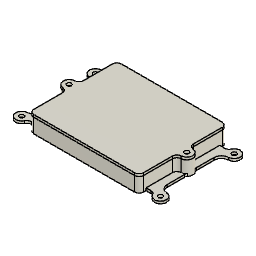
bat case v4 (Autodesk Fusion 360 design; units mm, degrees)
Autodesk Fusion 360 part; units mm, degrees
sketch "Sketch1" plane through (0, 0, 0) normal (0, 0, 1) x (1, 0, 0)
  line L0 (35.1, 27.7) -> (-35.1, 27.7)
  line L1 (-35.1, 27.7) -> (-35.1, -27.7)
  line L2 (-35.1, -27.7) -> (35.1, -27.7)
  line L3 (35.1, -27.7) -> (35.1, 27.7)
  line L4 (35.1, 27.7) -> (-35.1, -27.7) construction
  line L5 (-35.1, 27.7) -> (35.1, -27.7) construction
  circle A0 centre (-46.4, 24.65) radius 1.5
  circle A1 centre (-46.4, -24.65) radius 1.5
  line L6 (-40.0754, -24.65) -> (-36.7, -24.65)
  line L7 (-40.0754, 24.65) -> (-36.7, 24.65)
  arc A2 (-46.6015, -20.6551) -> (-42.786, -26.3643) centre (-46.4, -24.65) ccw
  arc A3 (-42.786, 26.3643) -> (-46.6015, 20.6551) centre (-46.4, 24.65) ccw
  arc A4 (-42.786, 26.3643) -> (-40.0754, 24.65) centre (-40.0754, 27.65) ccw
  arc A5 (-41.8533, 15.6614) -> (-46.6015, 20.6551) centre (-46.8533, 15.6614) ccw
  arc A6 (-46.6015, -20.6551) -> (-41.8533, -15.6614) centre (-46.8533, -15.6614) ccw
  arc A7 (-40.0754, -24.65) -> (-42.786, -26.3643) centre (-40.0754, -27.65) ccw
  line L8 (36.7, -29.3) -> (36.7, 29.3)
  line L9 (36.7, 29.3) -> (-36.7, 29.3)
  line L10 (-36.7, 29.3) -> (-36.7, -29.3)
  line L11 (-36.7, -29.3) -> (36.7, -29.3)
  line L12 (-36.7, 0) -> (-41.8533, 0) construction
  circle A8 centre (-39.2766, 0) radius 1.5
  line L13 (-41.8533, -15.6614) -> (-41.8533, -3.88)
  line L14 (-41.8533, 3.88) -> (-41.8533, 15.6614)
  arc A9 (-42.3277, 2.5867) -> (-42.3277, -2.5867) centre (-39.2766, 0) ccw
  arc A10 (-41.8533, -3.88) -> (-42.3277, -2.5867) centre (-43.8533, -3.88) ccw
  arc A11 (-42.3277, 2.5867) -> (-41.8533, 3.88) centre (-43.8533, 3.88) ccw
  dimension "d1" = 70.2
  dimension "d2" = 55.4
  dimension "d3" = 3
  dimension "d7" = 3
  dimension "d8" = 49.3
  dimension "d9" = 8
  dimension "d10" = 8
  dimension "d11" = 3
  dimension "d12" = 5
  dimension "d13" = 5
  dimension "d14" = 3
  dimension "d15" = 1.6
  dimension "d16" = 3
  dimension "d17" = 8
  dimension "d18" = 2
  dimension "d19" = 2
  constraint horizontal L0
  constraint perpendicular L0 L1
  constraint parallel L0 L2
  constraint parallel L1 L3
  constraint coincident L4 origin
  constraint coincident L5 origin
  constraint concentric A0 A3
  constraint concentric A1 A2
  constraint vertical L13
  constraint perpendicular L1 L6
  constraint perpendicular L1 L7
  constraint tangent L7 A4
  constraint tangent A3 A4
  constraint tangent A5 L13
  constraint tangent A3 A5
  constraint tangent A6 L13
  constraint tangent A2 A6
  constraint tangent L6 A7
  constraint tangent A2 A7
  constraint coincident L10 L7.end
  constraint coincident L10 L6.end
  constraint midpoint L10 L12.start
  constraint perpendicular L12 L13
  constraint midpoint L12 A8.centre
  constraint concentric A8 A9
  constraint collinear L13 L14
  constraint tangent L13 A10
  constraint tangent A9 A10
  constraint tangent L14 A11
  constraint tangent A9 A11
  measures "d1" distance of L1.end L2.end
  measures "d2" distance of L0.end L1.end
  measures "d3" diameter of A0
  measures "d7" diameter of A1
  measures "d8" distance of A0.centre A1.centre
  measures "d9" diameter of A3
  measures "d10" diameter of A2
  measures "d11" radius of A4
  measures "d12" radius of A5
  measures "d13" radius of A6
  measures "d14" radius of A7
  measures "d16" diameter of A8
  measures "d17" diameter of A9
  measures "d18" radius of A10
  measures "d19" radius of A11
extrude "Extrude1" add sketch "Sketch1" along normal blind 1.6 contours L0 L1 L2 L3 | A0 | A1 | L6 L7 A2 A3 A4 A5 A6 A7 L10 L13 L14 A9 A10 A11 | L8 L9 L10 L11 | A8 makes body 1
sketch "Sketch2" plane through (0, 0, 1.6) normal (0, 0, 1) x (-1, 0, 0)
  arc A0 (46.6015, 20.6551) -> (42.786, 26.3643) centre (46.4, 24.65) ccw
  arc A1 (40.0754, 24.65) -> (42.786, 26.3643) centre (40.0754, 27.65) ccw
  line L0 (40.0754, 24.65) -> (36.7, 24.65)
  line L1 (36.7, 24.65) -> (36.7, 29.3)
  line L2 (36.7, 29.3) -> (-36.7, 29.3)
  line L3 (-36.7, 29.3) -> (-36.7, -29.3)
  line L4 (-36.7, -29.3) -> (36.7, -29.3)
  line L5 (36.7, -29.3) -> (36.7, -24.65)
  line L6 (36.7, -24.65) -> (40.0754, -24.65)
  arc A2 (42.786, -26.3643) -> (40.0754, -24.65) centre (40.0754, -27.65) ccw
  arc A3 (42.786, -26.3643) -> (46.6015, -20.6551) centre (46.4, -24.65) ccw
  arc A4 (41.8533, -15.6614) -> (46.6015, -20.6551) centre (46.8533, -15.6614) ccw
  line L7 (41.8533, -15.6614) -> (41.8533, -3.88)
  arc A5 (42.3277, -2.5867) -> (41.8533, -3.88) centre (43.8533, -3.88) ccw
  arc A6 (42.3277, -2.5867) -> (42.3277, 2.5867) centre (39.2766, 0) ccw
  arc A7 (41.8533, 3.88) -> (42.3277, 2.5867) centre (43.8533, 3.88) ccw
  line L8 (41.8533, 3.88) -> (41.8533, 15.6614)
  arc A8 (46.6015, 20.6551) -> (41.8533, 15.6614) centre (46.8533, 15.6614) ccw
  line L9 (35.1, 27.7) -> (-35.1, 27.7)
  line L10 (35.1, -27.7) -> (35.1, 27.7)
  line L11 (-35.1, -27.7) -> (35.1, -27.7)
  line L12 (-35.1, 27.7) -> (-35.1, -27.7)
  line L13 (36.7, -29.3) -> (36.7, 29.3)
  line L14 (-36.7, -29.3) -> (36.7, -29.3)
  line L15 (-36.7, 29.3) -> (-36.7, -29.3)
  line L16 (36.7, 29.3) -> (-36.7, 29.3)
extrude "Extrude2" add sketch "Sketch2" along normal blind 8 contours L1 L2 L3 L4 L5 L13 L14 L15 L16 bodies 1
sketch "Sketch3" plane through (0, 0, 1.6) normal (0, 0, 1) x (-1, 0, 0)
  line L0 (36.7, 24.65) -> (36.7, -24.65)
  line L1 (36.7, -24.65) -> (40.0754, -24.65)
  arc A0 (42.786, -26.3643) -> (40.0754, -24.65) centre (40.0754, -27.65) ccw
  arc A1 (42.786, -26.3643) -> (46.6015, -20.6551) centre (46.4, -24.65) ccw
  arc A2 (41.8533, -15.6614) -> (46.6015, -20.6551) centre (46.8533, -15.6614) ccw
  line L2 (41.8533, -15.6614) -> (41.8533, -3.88)
  arc A3 (42.3277, -2.5867) -> (41.8533, -3.88) centre (43.8533, -3.88) ccw
  arc A4 (42.3277, -2.5867) -> (42.3277, 2.5867) centre (39.2766, 0) ccw
  arc A5 (41.8533, 3.88) -> (42.3277, 2.5867) centre (43.8533, 3.88) ccw
  line L3 (41.8533, 3.88) -> (41.8533, 15.6614)
  arc A6 (46.6015, 20.6551) -> (41.8533, 15.6614) centre (46.8533, 15.6614) ccw
  arc A7 (46.6015, 20.6551) -> (42.786, 26.3643) centre (46.4, 24.65) ccw
  arc A8 (40.0754, 24.65) -> (42.786, 26.3643) centre (40.0754, 27.65) ccw
  line L4 (40.0754, 24.65) -> (36.7, 24.65)
  circle A9 centre (46.4, 24.65) radius 1.5
  circle A10 centre (46.4, -24.65) radius 1.5
  circle A11 centre (39.2766, 0) radius 1.5
  arc A12 (36.7, -3.0596) -> (36.7, 3.0596) centre (39.2766, 0) ccw
  dimension "d30" = 8
  constraint concentric A11 A12
  constraint coincident L0 A12.end
  constraint coincident L0 A12.start
  measures "d30" diameter of A12
extrude "Extrude3" add sketch "Sketch3" along normal up to surface (8 mm away) contours L0 A4 A12 bodies 1
hole "Hole1" at (-46.4, 24.65, 1.6) direction (0, 0, -1) diameter 3 depth 10 tip angle 180 bodies 1
hole "Hole2" at (-46.4, -24.65, 1.6) direction (0, 0, -1) diameter 3 depth 10 tip angle 180 bodies 1
ref_plane "WorkPlane1" through (0, -16.1798, 4.8) normal (-1, 0, 0) x (0, -1, 0)
ref_plane "WorkPlane2" through (-36.7, -16.1798, 4.8) normal (-1, 0, 0) x (0, -1, 0)
split "Split1" by plane through (-36.7, -16.1798, 4.8) normal (-1, 0, 0) bodies 1 makes body 2 at (-38.4178, -1.2933, 0)
mirror "Mirror1" about plane through (0, -16.1798, 4.8) normal (-1, 0, 0) of bodies 2 makes body 3
ref_plane "WorkPlane3" through (0, 0, 9.6) normal (0, 0, 1) x (1, 0, 0)
sketch "Sketch4" plane through (0, 0, 9.6) normal (0, 0, 1) x (1, 0, 0)
  line L0 (-36.7, 29.3) -> (-36.7, -29.3)
  line L1 (-36.7, -29.3) -> (36.7, -29.3)
  line L2 (36.7, -29.3) -> (36.7, 29.3)
  line L3 (36.7, 29.3) -> (-36.7, 29.3)
  line L4 (35.1, 27.7) -> (35.1, -27.7)
  line L5 (35.1, -27.7) -> (-35.1, -27.7)
  line L6 (-35.1, -27.7) -> (-35.1, 27.7)
  line L7 (-35.1, 27.7) -> (35.1, 27.7)
  line L8 (-36.7, 29.3) -> (36.7, 29.3)
  line L9 (36.7, 29.3) -> (36.7, -29.3)
  line L10 (36.7, -29.3) -> (-36.7, -29.3)
  line L11 (-36.7, -29.3) -> (-36.7, 29.3)
  constraint horizontal L8
  constraint vertical L9
  constraint horizontal L10
  constraint vertical L11
  constraint coincident L1.end L2.start
  constraint coincident L0.start L3.end
extrude "Extrude4" add sketch "Sketch4" 2 faces at (37.0589, 0, 9.6) (-37.0589, 0, 9.6) along normal blind 1.6 separate body contours L0 L1 L2 L3 L8 L9 L10 L11 | L4 L5 L6 L7 on bodies 2 3 makes body 4
combine "Combine1" operation add target body 1 tool bodies 3 2
fillet "Fillet1" radius 3 8 edges at (36.7, -29.3, 4.8) (-36.7, -29.3, 4.8) (-36.7, 29.3, 4.8) (36.7, 29.3, 4.8) (36.7, -29.3, 10.4) (-36.7, -29.3, 10.4) (-36.7, 29.3, 10.4) (36.7, 29.3, 10.4) on bodies 1 4
fillet "Fillet2" radius 3 8 edges at (36.7, -3.0596, 5.6) (36.7, 3.0596, 5.6) (-36.7, 3.0596, 5.6) (-36.7, -3.0596, 5.6) (36.7, -3.0596, 10.4) (36.7, 3.0596, 10.4) (-36.7, 3.0596, 10.4) (-36.7, -3.0596, 10.4) on bodies 1 4
